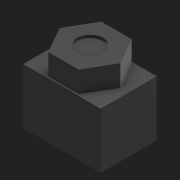
# Autodesk Inventor part: link_g0
Saved by Autodesk Inventor 2017 (Build 210142000, 142)
## iProperties
Created: 2019-08-03
Part Number: link_g0
Material: ABS Plastic
Document SubType Name: Modeling
Designer: Dell
Density: 1.06 g/cm^3
Appearance: Smooth - Black
Author: Dell
Autodesk Inventor part; units mm, degrees
ref_plane "YZ Plane" through (0, 0, 0) normal (1, 0, 0) x (0, 1, 0)
ref_plane "XZ Plane" through (0, 0, 0) normal (0, 1, 0) x (-1, 0, 0)
ref_plane "XY Plane" through (0, 0, 0) normal (0, 0, 1) x (1, 0, 0)
sketch "Sketch1" plane through (0, 0, 0) normal (0, 0, 1) x (1, 0, 0)
  line L0 (57.5, 0) -> (28.75, -49.7965)
  line L1 (28.75, -49.7965) -> (-28.75, -49.7965)
  line L2 (-28.75, -49.7965) -> (-57.5, 0)
  line L3 (-57.5, 0) -> (-28.75, 49.7965)
  line L4 (-28.75, 49.7965) -> (28.75, 49.7965)
  line L5 (28.75, 49.7965) -> (57.5, 0)
  point P0 (0, 0)
  point P1 (0, 0)
  dimension "d0" = 115
  constraints: 12 end point, 1 coincident, 1 horizontal alignment, 13 other
  measures "d0" distance of L0.start L2.end
extrude "Extrusion1" add sketch "Sketch1" along normal blind 40
sketch "Sketch2" plane through (0, 0, 0) normal (0, 0, -1) x (-1, 0, 0)
  line L0 (-73, 53) -> (73, 53)
  line L1 (73, 53) -> (73, -53)
  line L2 (73, -53) -> (-73, -53)
  line L3 (-73, -53) -> (-73, 53)
  point P0 (0, 0)
  point P1 (0, 53)
  point P2 (-73, 0)
  dimension "d3" = 146
  dimension "d4" = 106
  constraints: 8 end point, 2 midpoint, 2 parallel, 1 horizontal, 1 horizontal alignment, 1 perpendicular, 1 vertical alignment
  measures "d3" distance of L1.end L2.end
  measures "d4" distance of L0.end L1.end
extrude "Extrusion2" add sketch "Sketch2" along normal blind 105
sketch "Sketch3" plane through (0, 0, 40) normal (0, 0, 1) x (1, 0, 0)
  circle A0 centre (0, 0) radius 25
  dimension "d7" = 50
  constraints: 1 centre point, 1 coincident
  measures "d7" diameter of A0
extrude "Extrusion3" cut sketch "Sketch3" against normal blind 5
sketch "Sketch4" plane through (0, 0, -105) normal (0, 0, -1) x (-1, 0, 0)
  line L0 (56, 11.5) -> (-56, 11.5)
  line L1 (-56, 11.5) -> (-56, -11.5)
  line L2 (-56, -11.5) -> (56, -11.5)
  line L3 (56, -11.5) -> (56, 11.5)
  point P0 (0, 0)
  point P1 (56, 0)
  point P2 (0, 11.5)
  dimension "d10" = 23
  dimension "d11" = 112
  constraints: 8 end point, 2 midpoint, 2 parallel, 1 horizontal, 1 horizontal alignment, 1 perpendicular, 1 vertical alignment
  measures "d10" distance of L2.end L0.start
  measures "d11" distance of L1.end L2.end
extrude "Extrusion4" cut sketch "Sketch4" against normal blind 20
sketch "Sketch5" plane through (-56, -11.5, -105) normal (1, 0, 0) x (0, 0, -1)
  circle A0 centre (-10, 11.5) radius 2.5
  line L0 (0, 23) -> (0, 0) projected
  line L1 (0, 23) -> (-20, 23) projected
  line L2 (-20, 23) -> (-20, 0) projected
  line L3 (0, 0) -> (-20, 0) projected
  point P0 (-105, 11.5)
  point P1 (0, 11.5)
  point P2 (-10, 23)
  dimension "d14" = 5
  constraints: 2 midpoint, 1 centre point, 1 horizontal alignment, 1 vertical alignment
  measures "d14" diameter of A0
extrude "Extrusion5" cut sketch "Sketch5" along normal blind 117 and the other way blind 5 contours A0
body "Solid1"
